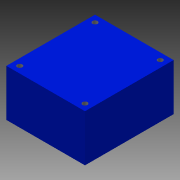
# Autodesk Inventor part: Motor board ver2
Saved by Autodesk Inventor 2015 (Build 190159000, 159)
## iProperties
Created: 2015-07-05
Part Number: Motor board ver2
Material: 一般
Document SubType Name: Modeling
Designer: kenta
Density: 1 g/cm^3
Appearance: 既定
Author: kenta
Autodesk Inventor part; units mm, degrees
ref_plane "YZ Plane" through (0, 0, 0) normal (1, 0, 0) x (0, 1, 0)
ref_plane "XZ Plane" through (0, 0, 0) normal (0, 1, 0) x (-1, 0, 0)
ref_plane "XY Plane" through (0, 0, 0) normal (0, 0, 1) x (1, 0, 0)
sketch "スケッチ1" plane through (0, 0, 0) normal (0, 0, 1) x (1, 0, 0)
  line L0 (-23.5, 26.5) -> (23.5, 26.5)
  line L1 (23.5, 26.5) -> (23.5, -26.5)
  line L2 (23.5, -26.5) -> (-23.5, -26.5)
  line L3 (-23.5, -26.5) -> (-23.5, 26.5)
  line L4 (-23.5, 26.5) -> (23.5, -26.5) construction
  line L5 (23.5, 26.5) -> (-23.5, -26.5) construction
  point P0 (0, 0)
  dimension "d0" = 47
  dimension "d1" = 53
  constraints: 12 end point, 2 midpoint, 2 parallel, 1 horizontal, 1 perpendicular
  measures "d0" distance of L1.end L2.end
  measures "d1" distance of L0.end L1.end
extrude "押し出し1" add sketch "スケッチ1" along normal blind 28
sketch "スケッチ2" plane through (0, 0, 0) normal (0, 0, -1) x (-1, 0, 0)
  line L0 (23.5, -26.5) -> (23.5, 26.5) projected
  line L1 (23.5, -26.5) -> (-23.5, -26.5) projected
  line L2 (23.5, 26.5) -> (-23.5, 26.5) projected
  line L3 (-23.5, 26.5) -> (-23.5, -26.5) projected
  point P0 (0, 0)
  point P1 (19.5, -22.5)
  point P2 (19.5, 22.5)
  point P3 (-19.5, 22.5)
  point P4 (-19.5, -22.5)
  dimension "d4" = 4
  dimension "d5" = 4
  dimension "d6" = 4
  dimension "d7" = 4
  constraints: 2 horizontal alignment, 2 vertical alignment
  measures "d4" distance from line of point (19.5, -22.5) L0
  measures "d5" distance from line of L1 point (19.5, -22.5)
  measures "d6" distance from line of point (19.5, 22.5) L2
  measures "d7" distance from line of point (-19.5, 22.5) L3
hole "穴1" at (-19.5, -22.5, 0) at (-19.5, 22.5, 0) at (19.5, 22.5, 0) at (19.5, -22.5, 0) direction (0, 0, 1) diameter 3 end through all
